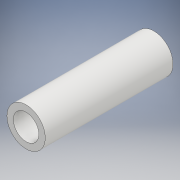
# Autodesk Inventor part: tube
Saved by Autodesk Inventor 2017.3 (Build 213256000, 256)
## iProperties
Part Number: tube
Material: Tuyauterie PVC
Document SubType Name: Modeling
Designer: Piou piou
Density: 1.4 g/cm^3
Appearance: Lisse - Blanc
Mass: 6.87223 g
Surface Area: 41.2334 cm^2
Volume: 4.90874 cm^3
Author: Piou piou
Autodesk Inventor part; units mm, degrees
ref_plane "YZ Plane" through (0, 0, 0) normal (1, 0, 0) x (0, 1, 0)
ref_plane "XZ Plane" through (0, 0, 0) normal (0, 1, 0) x (-1, 0, 0)
ref_plane "XY Plane" through (0, 0, 0) normal (0, 0, 1) x (1, 0, 0)
sketch "Esquisse1" plane through (0, 0, 0) normal (0, 1, 0) x (-1, 0, 0)
  circle A0 centre (0, 0) radius 7.5
  circle A1 centre (0, 0) radius 5
  dimension "d0" = 15
  dimension "d1" = 10
  constraints: 2 centre point, 2 coincident
  measures "d0" diameter of A0
  measures "d1" diameter of A1
extrude "Extrusion1" add sketch "Esquisse1" along normal blind 50
